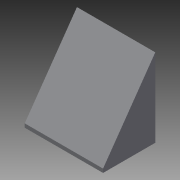
# Autodesk Inventor part: Slave Tablet Angle Wedge 35 Degrees
Saved by Autodesk Inventor 2014 SP2 (Build 180246200, 246)
## iProperties
Created: 2015-08-04
Part Number: Slave Tablet Angle Wedge 35 Degrees
Material: Generic
Document SubType Name: Modeling
Designer: Devon
Density: 1 g/cm^3
Appearance: Default
Author: Devon
Autodesk Inventor part; units mm, degrees
ref_plane "YZ Plane" through (0, 0, 0) normal (1, 0, 0) x (0, 1, 0)
ref_plane "XZ Plane" through (0, 0, 0) normal (0, 1, 0) x (-1, 0, 0)
ref_plane "XY Plane" through (0, 0, 0) normal (0, 0, 1) x (1, 0, 0)
sketch "Sketch1" plane through (0, 0, 0) normal (0, 0, 1) x (1, 0, 0)
  line L0 (19.7632, 4.9157) -> (57.8632, 4.9157)
  line L1 (57.8632, 4.9157) -> (57.8632, -33.1843)
  line L2 (57.8632, -33.1843) -> (19.7632, -33.1843)
  line L3 (19.7632, -33.1843) -> (19.7632, 4.9157)
  point P0 (0, 0)
  dimension "d0" = 38.1
  dimension "d1" = 38.1
  constraints: 8 end point, 2 parallel, 1 horizontal, 1 perpendicular
  measures "d0" distance of L1.end L2.end
  measures "d1" distance of L0.end L1.end
extrude "Extrusion1" add sketch "Sketch1" along normal blind 25.4
sketch "Sketch2" plane through (57.8632, -33.1843, 0) normal (1, 0, 0) x (0, 0, -1)
  line L0 (0, 38.1) -> (-27.0968, -0.5982)
  line L1 (0, 38.1) -> (47.2418, 38.1) construction
  point P0 (0, 33.1843)
  dimension "d4" = 125
  constraints: 4 end point, 1 equal length, 1 horizontal
  measures "d4" angle of L0 L1
split body "Split1" sketch "Sketch2" result one side removed curves L0 removed pieces at (32.4632, -6.8891, 8.8762)
body "Solid1"
